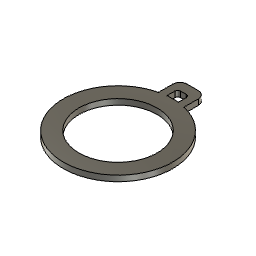
Flag Pole Ring (Autodesk Fusion 360 design; units mm, degrees)
Autodesk Fusion 360 part; units mm, degrees
sketch "Sketch1" plane through (0, 0, 0) normal (0, 0, 1) x (1, 0, 0)
  circle A0 centre (0, 0) radius 19.25
  circle A1 centre (0, 0) radius 13.725
  line L0 (0, 0) -> (4.5, 0)
  line L1 (4.5, 0) -> (4.5, 19.25)
  line L2 (4.5, 19.25) -> (0, 19.25)
  line L3 (0, 19.25) -> (0, 0)
  line L4 (0, 0) -> (-4.5, 0)
  line L5 (-4.5, 0) -> (-4.5, 19.25)
  line L6 (-4.5, 19.25) -> (0, 19.25)
  line L7 (0, 19.25) -> (0, 0)
  line L8 (4.5, 19.25) -> (-4.5, 19.25)
  line L9 (-4.5, 19.25) -> (-4.5, 26.25)
  line L10 (-4.5, 26.25) -> (4.5, 26.25)
  line L11 (4.5, 26.25) -> (4.5, 19.25)
  line L12 (0, 19.25) -> (2, 19.25)
  line L13 (2, 19.25) -> (2, 23)
  line L14 (2, 23) -> (0, 23)
  line L15 (0, 23) -> (0, 19.25)
  line L16 (0, 19.25) -> (-2, 19.25)
  line L17 (-2, 19.25) -> (-2, 23)
  line L18 (-2, 23) -> (0, 23)
  line L19 (0, 23) -> (0, 19.25)
  dimension "d1" = 38.5
  dimension "d2" = 27.45
  dimension "d3" = 4.5
  dimension "d4" = 19.25
  dimension "d5" = 4.5
  dimension "d6" = 19.25
  dimension "d7" = 7
  constraint coincident A0.centre A1.centre
  constraint concentric A0 A1
  constraint horizontal L0
  constraint vertical L1
  constraint horizontal L2
  constraint vertical L3
  constraint horizontal L4
  constraint vertical L5
  constraint horizontal L6
  constraint vertical L7
  constraint horizontal L8
  constraint vertical L9
  constraint horizontal L10
  constraint vertical L11
  constraint horizontal L12
  constraint vertical L13
  constraint horizontal L14
  constraint vertical L15
  constraint horizontal L16
  constraint vertical L17
  constraint horizontal L18
  constraint vertical L19
  measures "d1" diameter of A0
  measures "d2" diameter of A1
  measures "d3" distance of A0.centre L0.end
  measures "d4" distance of A0.centre L2.end
  measures "d5" distance of A0.centre L4.end
  measures "d6" distance of A0.centre L2.end
  measures "d7" distance of L1.end L10.end
extrude "Extrude1" add sketch "Sketch1" along normal blind 2 contours A0 A1 L1 L5 | A0 A1 L1 L3 L7 | A0 L1 L2 L8 L12 | A0 L5 L6 L8 L16 | A0 A1 L3 L5 L7 | L2 L6 L8 L9 L10 L11 L13 L14 L17 L18
fillet "Fillet1" radius 1 1 edges at (-2, 23, 1)
fillet "Fillet2" radius 1 1 edges at (2, 23, 1)
fillet "Fillet3" radius 2.5 1 edges at (-4.5, 26.25, 1)
fillet "Fillet4" radius 2.5 1 edges at (4.5, 26.25, 1)
